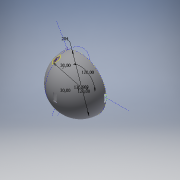
# Autodesk Inventor part: Schale_V1
Saved by Autodesk Inventor 2017 (Build 210142000, 142)
## iProperties
Part Number: Schale_V1
Material: Generisch
Document SubType Name: Modeling
Designer: Enno-LT
Density: 1 g/cm^3
Appearance: Vorgabe
Author: Enno-LT
Autodesk Inventor part; units mm, degrees
ref_plane "YZ Plane" through (0, 0, 0) normal (1, 0, 0) x (0, 1, 0)
ref_plane "XZ Plane" through (0, 0, 0) normal (0, 1, 0) x (-1, 0, 0)
sketch "Skizze2" plane through (0, 0, 0) normal (0, 0, 1) x (1, 0, 0)
  line L0 (100, 0) -> (102, 0)
  arc A0 (0, -102) -> (102, 0) centre (0, 0) ccw
  line L1 (0, -102) -> (0, -100)
  arc A1 (0, -100) -> (100, 0) centre (0, 0) ccw
  point P0 (0, 0)
  point P1 (0, -101)
  point P2 (101, 0)
  dimension "d0" = 2
  dimension "d1" = 2
  dimension "d3" = 100
  dimension "d4" = 100
  constraints: 4 end point, 4 point on circle, 2 centre point, 2 midpoint, 2 point on line, 2 vertical alignment, 1 horizontal, 1 horizontal alignment, 1 perpendicular
  measures "d0" distance of L0.start L0.end
  measures "d1" distance of L1.start L1.end
  measures "d3" distance of point (0, 0) L1.end
  measures "d4" horizontal distance of L0.start point (0, -101)
revolve "Umdrehung1" add sketch "Skizze2" angle 360 about axis through (0, -102, 0) along (0, 1, 0)
ref_plane "Arbeitsebene1" through (0, -102, 0) normal (0, 1, 0) x (-1, 0, 0)
sketch "Skizze3" plane through (0, -102, 0) normal (0, 1, 0) x (-1, 0, 0)
  line L0 (7.5, 15) -> (-7.5, 15)
  line L1 (-7.5, 15) -> (-7.5, -15)
  line L2 (-7.5, -15) -> (7.5, -15)
  line L3 (7.5, -15) -> (7.5, 15)
  point P0 (0, 0)
  point P1 (7.5, 0)
  point P2 (0, 15)
  dimension "d6" = 15
  dimension "d7" = 30
  constraints: 8 end point, 2 midpoint, 2 parallel, 1 horizontal, 1 horizontal alignment, 1 perpendicular, 1 vertical alignment
  measures "d6" distance of L1.end L2.end
  measures "d7" distance of L0.end L1.end
extrude "Extrusion1" cut sketch "Skizze3" along normal through all both and the other way through all
sketch "Skizze4" plane through (0, 0, 0) normal (1, 0, 0) x (0, 1, 0)
  line L0 (7.5, 15) -> (-7.5, 15)
  line L1 (-7.5, 15) -> (-7.5, -15)
  line L2 (-7.5, -15) -> (7.5, -15)
  line L3 (7.5, -15) -> (7.5, 15)
  point P0 (0, 0)
  point P1 (0, 0)
  point P2 (7.5, 0)
  point P3 (0, 15)
  point P4 (-7.5, 0)
  dimension "d10" = 15
  dimension "d11" = 30
  constraints: 8 end point, 3 midpoint, 2 horizontal alignment, 2 parallel, 2 vertical alignment, 1 horizontal, 1 perpendicular
  measures "d10" distance of L1.end L2.end
  measures "d11" distance of L0.end L1.end
extrude "Extrusion2" cut sketch "Skizze4" along normal through all
sketch "Skizze6" plane through (0, 0, 0) normal (0, 1, 0) x (1, 0, 0)
  line L0 (0, 0) -> (-94.1178, 163.0168) construction
  line L1 (0, 0) -> (188.2356, 0) construction
  line L2 (0, 0) -> (-95.3588, -165.1662) construction
  line L3 (0, 0) -> (190.7175, 0) construction
  arc A0 (100.891, 15) -> (100.891, -15) centre (0, 0) ccw construction
  point P0 (-51, -88.3346)
  point P1 (-51, 88.3346)
  dimension "d16" = 120
  dimension "d17" = 120
  constraints: 8 end point, 2 equal length, 2 horizontal, 2 point on circle, 2 point on line
  measures "d16" angle of L1 L0
  measures "d17" angle of L2 L3
ref_plane "Arbeitsebene7" through (-51, 0, -88.3346) normal (1, 0, 0) x (0, 1, 0)
sketch "Skizze14" plane through (-51, 0, -88.3346) normal (1, 0, 0) x (0, 1, 0)
  circle A0 centre (0, 88.3346) radius 88.3346 construction
  line L0 (0, 88.3346) -> (-48.5836, 172.4838) construction
  line L1 (0, 188.3346) -> (0, -11.6654) construction
  line L2 (0, 88.3346) -> (-62.5691, -20.0382) construction
  point P0 (0, 103.3346)
  point P1 (0, 73.3346)
  point P2 (-44.1673, 164.8346)
  point P3 (-44.1673, 11.8346)
  dimension "d38" = 176.6692
  dimension "d39" = 30
  dimension "d40" = 30
  constraints: 4 end point, 2 point on circle, 2 point on line, 1 centre point, 1 coincident
  measures "d38" diameter of A0
  measures "d39" angle of L1 L0
  measures "d40" angle of L1 L2
sketch "Skizze16" plane through (0, 0, 0) normal (0, 1, 0) x (1, 0, 0)
  circle A0 centre (0, 0) radius 102 construction
  arc A1 (100.891, 15) -> (100.891, -15) centre (0, 0) ccw construction
  arc A2 (100.6119, -15) -> (100.6119, 15) centre (0, 0) ccw construction
  point P0 (101.7239, 0)
  dimension "d37" = 204
  constraints: 1 centre point, 1 coincident, 1 concentric, 1 point on circle
  measures "d37" diameter of A0
ref_plane "Arbeitsebene8" through (-51, -44.1673, -76.5) normal (-0.5, -0.433, -0.75) x (0.6547, -0.7559, 0)
ref_plane "Arbeitsebene9" through (-51, -44.1673, 76.5) normal (-0.5, -0.433, 0.75) x (0.6547, -0.7559, 0)
sketch "Skizze17" plane through (-51, -44.1673, -76.5) normal (-0.5, -0.433, -0.75) x (0.6547, -0.7559, 0)
  point P0 (0, 0)
  point P1 (0, 0)
  constraints: 1 coincident
hole "Bohrung3" at (-51, -44.1673, -76.5) direction (0.5, 0.433, 0.75) diameter 21 depth 8 tip angle 118
sketch "Skizze18" plane through (-51, -44.1673, 76.5) normal (-0.5, -0.433, 0.75) x (0.6547, -0.7559, 0)
  point P0 (0, 0)
  point P1 (0, 0)
  constraints: 1 coincident
hole "Bohrung4" at (-51, -44.1673, 76.5) direction (0.5, 0.433, -0.75) diameter 21 depth 8 tip angle 118
